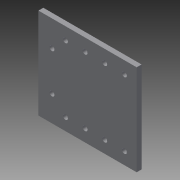
# Autodesk Inventor part: AX12_gabarit
Saved by Autodesk Inventor 2014 (Build 180170000, 170)
## iProperties
Created: 2014-01-10
Part Number: AX12_gabarit
Material: Générique
Document SubType Name: Modeling
Designer: helly
Density: 1 g/cm^3
Appearance: Par défaut
Author: helly
Autodesk Inventor part; units mm, degrees
ref_plane "YZ Plane" through (0, 0, 0) normal (1, 0, 0) x (0, 1, 0)
ref_plane "XZ Plane" through (0, 0, 0) normal (0, 1, 0) x (-1, 0, 0)
ref_plane "XY Plane" through (0, 0, 0) normal (0, 0, 1) x (1, 0, 0)
sketch "Esquisse1" plane through (0, 0, 0) normal (0, 1, 0) x (-1, 0, 0)
  line L0 (0, 0) -> (0, 27) construction
  line L1 (0, 0) -> (24, 0) construction
  line L2 (24, 0) -> (24, 27) construction
  line L3 (24, 27) -> (0, 27) construction
  line L4 (0, 0) -> (8, 0) construction
  line L5 (8, 0) -> (16, 0) construction
  line L6 (16, 0) -> (24, 0) construction
  circle A0 centre (0, 0) radius 1
  circle A1 centre (8, 0) radius 1
  circle A2 centre (16, 0) radius 1
  circle A3 centre (24, 0) radius 1
  line L7 (24, 0) -> (29.5, 0) construction
  circle A4 centre (0, 27) radius 1
  circle A5 centre (8, 27) radius 1
  circle A6 centre (16, 27) radius 1
  circle A7 centre (24, 27) radius 1
  line L8 (29.5, 0) -> (29.5, 5.5) construction
  line L9 (29.5, 5.5) -> (29.5, 21.5) construction
  circle A8 centre (29.5, 21.5) radius 1
  circle A9 centre (29.5, 5.5) radius 1
  line L10 (0, 0) -> (0, -5) construction
  line L11 (0, -5) -> (-5, -5) construction
  line L12 (-5, -5) -> (-5, 32)
  line L13 (-5, 32) -> (35, 32)
  line L14 (35, 32) -> (35, -5)
  line L15 (35, -5) -> (-5, -5)
  line L16 (16, 0) -> (24, 0) construction
  dimension "d0" = 8
  dimension "d1" = 8
  dimension "d2" = 2
  dimension "d3" = 2
  dimension "d4" = 5.5
  dimension "d5" = 2
  dimension "d6" = 2
  dimension "d7" = 5.5
  dimension "d8" = 16
  dimension "d9" = 2
  dimension "d10" = 2
  dimension "d12" = 27
  dimension "d13" = 5
  dimension "d15" = 8
  dimension "d16" = 5.5
  dimension "d17" = 40
  dimension "d18" = 32
  dimension "d19" = 19
  dimension "d20" = 27
  constraints: 34 end point, 10 centre point, 8 coincident, 6 perpendicular, 4 collinear, 4 equal radius, 4 parallel, 4 point on line, 1 vertical
  measures "d0" distance of L0.start L4.end
  measures "d1" distance of L4.end L5.end
  measures "d2" diameter of A1
  measures "d3" diameter of A2
  measures "d4" distance of L7.start L7.end
  measures "d5" diameter of A4
  measures "d6" diameter of A5
  measures "d7" distance of L7.end L8.end
  measures "d8" distance of L8.end L9.end
  measures "d9" diameter of A8
  measures "d10" diameter of A9
  measures "d12" distance of L0.start L0.end
  measures "d13" distance of L10.start L10.end
  measures "d15" distance of L16.start L7.start
  measures "d16" distance between parallel lines of L8 L14
  measures "d17" distance between parallel lines of L14 L12
  measures "d18" distance between parallel lines of L7 L13
  measures "d19" distance from line of A6.centre L14
  measures "d20" distance from line of A5.centre L14
extrude "Extrusion1" add sketch "Esquisse1" along normal blind 2
